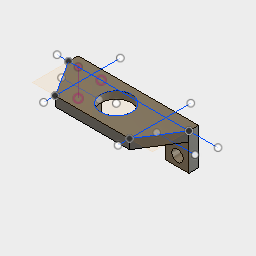
encoder-bracket (Autodesk Fusion 360 design; units mm, degrees)
Autodesk Fusion 360 part; units mm, degrees
box "BoxPrimitive1" add length 15.24 width 39.878 height 3.175 placed x (0, 0, 1) y (1, 0, 0) z (0, 1, 0) at (0, 0, 0)
sketch "Sketch3" plane through (0, 3.175, 0) normal (0, 1, 0) x (-1, 0, 0)
  line L0 (0, 15.24) -> (-39.878, 15.24)
  line L1 (-39.878, 15.24) -> (-39.878, 0)
  line L2 (-39.878, 0) -> (0, 0)
  line L3 (0, 0) -> (0, 15.24)
  circle A0 centre (-19.939, 7.3025) radius 5.08
  line L4 (3.81, 3.175) -> (-49.53, 3.175)
  line L5 (-7.62, -6.35) -> (-7.62, 19.05)
  line L6 (0, 3.175) -> (-7.62, 15.24)
  line L7 (-32.258, -5.08) -> (-32.258, 19.0381)
  line L8 (-32.258, 15.24) -> (-39.878, 3.175)
  dimension "d6" = 10.16
  dimension "d7" = 19.939
  dimension "d8" = 7.3025
  dimension "d15" = 3.175
  dimension "d16" = 7.62
  dimension "d17" = 7.62
  measures "d6" diameter of A0
  measures "d7" distance of L3 A0.centre
  measures "d8" distance of L2 A0.centre
  measures "d15" distance of L2.end L4.start
  measures "d16" distance of L2.end L5.start
  measures "d17" distance of L1.end L7.start
hole "Hole1" at (19.939, 0, 7.3025) direction (0, 1, 0) diameter 10.16 depth 10.16 tip angle 90 counterbore diameter 12.7 counterbore depth 0.762
extrude "Extrude1" cut sketch "Sketch3" against normal blind 3.175 contours L0 L3 L6
extrude "Extrude2" cut sketch "Sketch3" against normal blind 3.175 contours L0 L1 L8
box "BoxPrimitive2" add length 9.017 width 7.62 height 3.175 placed x (0, -1, 0) y (1, 0, 0) z (0, 0, 1) at (0, 0, 0)
hole "Hole2" at (3.81, -5.842, 3.175) direction (0, 0, -1) diameter 3.81 depth 3.175 tip angle 180
box "BoxPrimitive3" add length 9.017 width 7.62 height 3.175 placed x (0, -1, 0) y (1, 0, 0) z (0, 0, 1) at (32.258, 0, 0)
hole "Hole3" at (36.068, -5.842, 3.175) direction (0, 0, -1) diameter 3.81 depth 3.175 tip angle 180
sketch "Sketch6" plane through (0, 0, 0) normal (0, 0, 1) x (1, 0, 0)
  line L0 (7.62, 0) -> (0, 0)
  line L1 (0, 0) -> (0, -9.017)
sketch "Sketch7" plane through (0, 0, 3.175) normal (0, 0, 1) x (1, 0, 0)
  circle A0 centre (3.81, -5.842) radius 1.905
  line L0 (0, -9.017) -> (7.62, -9.017)
  line L1 (7.62, -9.017) -> (7.62, 0)
  line L2 (7.62, 0) -> (0, 0)
  line L3 (0, 0) -> (0, -9.017)
  line L4 (-2.286, -2.667) -> (10.16, -2.667)
  dimension "d40" = 6.35
  measures "d40" distance of L0 L4.end
sketch "Sketch8" plane through (0, 0, 3.175) normal (0, 0, 1) x (1, 0, 0)
  circle A0 centre (36.068, -5.842) radius 1.905
  line L0 (32.258, -9.017) -> (39.878, -9.017)
  line L1 (39.878, -9.017) -> (39.878, 0)
  line L2 (39.878, 0) -> (32.258, 0)
  line L3 (32.258, 0) -> (32.258, -9.017)
  line L4 (29.21, -2.667) -> (41.91, -2.667)
  dimension "d43" = 6.35
  measures "d43" distance of L0 L4.end
sketch "Sketch9" plane through (0, 0, 0) normal (0, -1, 0) x (1, 0, 0)
  line L0 (32.258, 3.175) -> (39.878, 3.175)
  line L1 (39.878, 3.175) -> (32.258, 15.24)
  line L2 (32.258, 15.24) -> (7.62, 15.24)
  line L3 (7.62, 15.24) -> (0, 3.175)
  line L4 (0, 3.175) -> (7.62, 3.175)
  line L5 (7.62, 3.175) -> (7.62, 0)
  line L6 (7.62, 0) -> (32.258, 0)
  line L7 (32.258, 0) -> (32.258, 3.175)
  circle A0 centre (19.939, 7.3025) radius 6.35
  line L8 (19.939, 7.3025) -> (19.939, 21.5253)
  line L9 (30.099, 20.32) -> (30.099, -2.54)
  line L10 (19.939, 7.3025) -> (43.18, 7.3025)
  line L11 (31.369, 5.3975) -> (28.829, 5.3975)
  line L12 (28.829, 5.3975) -> (28.829, 9.2075)
  line L13 (28.829, 9.2075) -> (31.369, 9.2075)
  line L14 (31.369, 9.2075) -> (31.369, 5.3975)
  line L15 (31.369, 5.3975) -> (28.829, 9.2075) construction
  line L16 (28.829, 5.3975) -> (31.369, 9.2075) construction
  point P0 (30.099, 7.3025)
  dimension "d46" = 10.16
  dimension "d47" = 3.81
  dimension "d48" = 2.54
  measures "d46" distance of L8 L9
  measures "d47" distance of L11 L13
  measures "d48" distance of L12 L14
extrude "Extrude5" cut sketch "Sketch9" against normal blind 1.905 contours L9 L10 L11 L14 | L9 L10 L13 L14 | L9 L10 L11 L12 | L9 L10 L12 L13
